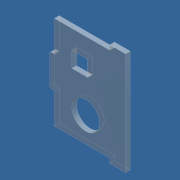
# Autodesk Inventor part: Back_plate
Saved by Autodesk Inventor 2016 (Build 200138000, 138)
## iProperties
Created: 2016-04-04
Part Number: Back_plate
Material: Polycarbonate, Clear
Document SubType Name: Modeling
Designer: admin
Density: 1.2 g/cm^3
Appearance: Polycarbonate - Clear
Author: admin
Autodesk Inventor part; units mm, degrees
ref_plane "YZ Plane" through (0, 0, 0) normal (1, 0, 0) x (0, 1, 0)
ref_plane "XZ Plane" through (0, 0, 0) normal (0, 1, 0) x (-1, 0, 0)
ref_plane "XY Plane" through (0, 0, 0) normal (0, 0, 1) x (1, 0, 0)
derived "Fan_plate.ipt"
sketch "Sketch1" plane through (0, 0, 0) normal (0, 1, 0) x (-1, 0, 0)
  line L0 (17.5, -29.5) -> (-17.5, -29.5)
  line L1 (-17.5, -29.5) -> (-17.5, -32.5)
  line L2 (-17.5, -32.5) -> (-27.5, -32.5)
  line L3 (-27.5, -32.5) -> (-27.5, 32.5)
  line L4 (-27.5, 32.5) -> (-17.5, 32.5)
  line L5 (-17.5, 32.5) -> (-17.5, 29.5)
  line L6 (-17.5, 29.5) -> (17.5, 29.5)
  line L7 (17.5, -10) -> (19.5, -10)
  line L8 (20.5, -9) -> (20.5, 9)
  line L9 (19.5, 10) -> (17.5, 10)
  line L10 (17.5, 29.5) -> (17.5, 10)
  line L11 (17.5, -10) -> (17.5, -29.5)
  arc A0 (20.5, 9) -> (19.5, 10) centre (19.5, 9) ccw
  arc A1 (19.5, -10) -> (20.5, -9) centre (19.5, -9) ccw
  point P0 (0, 0)
  point P1 (-27.5, 0)
  point P2 (0, -29.5)
  point P3 (20.5, 0)
extrude "Extrusion1" add sketch "Sketch1" along normal blind 3
sketch "Sketch2" plane through (-17.5, 0, -29.5) normal (0, -1, 0) x (1, 0, 0)
  circle A0 centre (19.746, 15.7634) radius 8.746
  line L0 (21, 47.1318) -> (11, 47.1318)
  line L1 (11, 47.1318) -> (11, 37.1318)
  line L2 (11, 37.1318) -> (21, 37.1318)
  line L3 (21, 37.1318) -> (21, 47.1318)
  line L4 (0, 39.5) -> (0, 59) projected
  point P0 (17.5, 29.5)
  dimension "d3" = 11
  dimension "d4" = 10
  constraints: 8 end point, 2 parallel, 2 perpendicular, 1 centre point, 1 horizontal, 1 tangent
  measures "d3" distance between parallel lines of L4 L1
  measures "d4" distance of L0.start L0.end
extrude "Extrusion2" cut sketch "Sketch2" against normal blind 10
body "Solid1"
